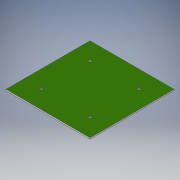
# Autodesk Inventor part: PCB_sheald
Saved by Autodesk Inventor 2019 (Build 230136000, 136)
## iProperties
Created: 2023-04-17
Part Number: PCB_sheald
Material: Generic
Document SubType Name: Sheet Metal
Designer: Analuam
Density: 1 g/cm^3
Sheet Metal Rule: Default_mm
Appearance: Default
Author: Analuam
Autodesk Inventor part; units mm, degrees
ref_plane "YZ Plane" through (0, 0, 0) normal (1, 0, 0) x (0, 1, 0)
ref_plane "XZ Plane" through (0, 0, 0) normal (0, 1, 0) x (-1, 0, 0)
ref_plane "XY Plane" through (0, 0, 0) normal (0, 0, 1) x (1, 0, 0)
sketch "Sketch1" plane through (0, 0, 0) normal (0, 1, 0) x (-1, 0, 0)
  line L0 (7.6649, 9.6125) -> (-92.3351, 9.6125)
  line L1 (-92.3351, 9.6125) -> (-92.3351, -90.3875)
  line L2 (-92.3351, -90.3875) -> (7.6649, -90.3875)
  line L3 (7.6649, -90.3875) -> (7.6649, 9.6125)
  circle A0 centre (-13.4287, -11.481) radius 1.5
  circle A1 centre (-13.4287, -69.294) radius 1.5
  circle A2 centre (-71.2416, -11.481) radius 1.5
  circle A3 centre (-71.2416, -69.294) radius 1.5
  point P0 (0, 0)
  point P1 (-71.2417, -69.294)
  point P2 (-71.2417, -11.481)
  point P3 (-13.4287, -69.294)
  dimension "d0" = 100
  dimension "d1" = 100
  dimension "d2" = 57.813
  dimension "d3" = 57.813
  dimension "d4" = 3
  constraints: 8 end point, 4 centre point, 2 parallel, 1 coincident, 1 horizontal, 1 perpendicular
  measures "d0" distance of L2.end L1.end
  measures "d1" distance of L1.end L0.end
  measures "d2" distance of point (-13.429, -69.294) point (-71.242, -69.294)
  measures "d3" distance of point (-71.242, -69.294) point (-71.242, -11.481)
  measures "d4" diameter of A0
extrude "Extrusion1" add sketch "Sketch1" along normal blind 1.5
equation "\"BendRadius\" = Thickness"
equation "\"BendReliefWidth\" = Thickness"
equation "\"BendReliefDepth\" = 0.5 * Thickness"
equation "\"CornerReliefSize\" = 4 * Thickness"
equation "\"MinimumRemnant\" = 2 * Thickness"
equation "\"TransitionRadius\" = BendRadius"
equation "\"JacobiRadiusSize\" = BendRadius"
equation "\"GapSize\" = Thickness"
equation "\"Thickness\" = 0.5"
body "Solid1"
